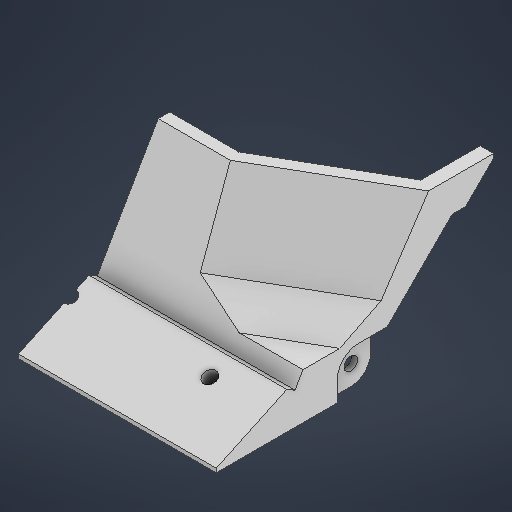
# Autodesk Inventor part: BodyFront
Saved by Autodesk Inventor 2027 (Build 310192000, 192)
## iProperties
Created: 2026-09-17
Part Number: BodyFront
Material: Všeobecné
Document SubType Name: Modeling
Designer: Vadim
Density: 1 g/cm^3
Appearance: Výchozí
Author: Vadim
Autodesk Inventor part; units mm, degrees
ref_plane "YZ Plane" through (0, 0, 0) normal (1, 0, 0) x (0, 1, 0)
ref_plane "XZ Plane" through (0, 0, 0) normal (0, 1, 0) x (-1, 0, 0)
ref_plane "XY Plane" through (0, 0, 0) normal (0, 0, 1) x (1, 0, 0)
sketch "Náčrt1" plane through (0, 0, 0) normal (1, 0, 0) x (0, 1, 0)
  circle A0 centre (0, 0) radius 5
  line L0 (5, 0) -> (5, -7)
  line L1 (5, -7) -> (21.5, -23.5)
  circle A1 centre (10.5, -45) radius 19.6
  circle A2 centre (8, -45) radius 19.6
  line L2 (21.5, -23.5) -> (21.5, -28.7778)
  line L3 (21.5, -28.2814) -> (29.5, -36.2814)
  circle A3 centre (10.5, -45) radius 18
  line L4 (28.5, -41.2264) -> (28.5, -45)
  line L5 (28.5, -41.2264) -> (28.1, -41.2264)
  line L6 (21.5, -26.8672) -> (29.5, -34.8672)
  line L7 (28.5, -41.2264) -> (29.5, -41.2264)
  line L8 (29.5, -41.2264) -> (29.5, -33.8672)
  line L9 (29.5, -33.8672) -> (28.5, -33.8672)
  line L10 (28.5, -33.8672) -> (28.5, -41.2264)
  line L11 (-5, 0) -> (-5, 35.5203)
  line L12 (7.6785, 17.8108) -> (-5, 45) construction
  line L13 (-5, 37.6648) -> (4.869, 16.5006) construction
  line L14 (4.869, 16.5006) -> (7.6785, 17.8108) construction
  line L15 (-5, 45) -> (-5, 37.6648) construction
  line L16 (-5, 35.5203) -> (-4, 35.5203)
  line L17 (-4, 35.5203) -> (4.2351, 17.8601)
  line L18 (29.5, 20.4961) -> (29.5, -33.8672)
  arc A4 (5.25, 0) -> (-5, 1.6008) centre (0, 0) ccw
  line L19 (5.25, 0) -> (5.25, -7.25)
  line L20 (4.2351, 17.8601) -> (3.0549, 15.816)
  line L21 (3.0549, 15.816) -> (29.5, 0.5479)
  line L22 (29.5, -2.3389) -> (-5, 17.5797)
  line L23 (5.25, 0) -> (5.25, 14.5486)
  line L24 (0, -5) -> (5, -5)
  line L25 (5, -5) -> (5.25, -5)
  line L26 (0, 5.25) -> (-5, 5.25)
  point P0 (5.25, 11.6619)
  dimension "d7" = 39.2
  dimension "d0" = 10
  dimension "d1" = 7
  dimension "d3" = 26.5
  dimension "d4" = 45
  dimension "d6" = 2.5
  dimension "d8" = 39.2
  dimension "d12" = 13
  dimension "d13" = 1.6
  dimension "d15" = 0.4
  dimension "d16" = 1
  dimension "d17" = 1
  dimension "d22" = 3.1
  dimension "d23" = 25
  dimension "d24" = 30
  dimension "d26" = 1
  dimension "d27" = 1.5
  dimension "d34" = 0.25
  dimension "d35" = 45
  dimension "d36" = 45
  dimension "d39" = 1.5
  dimension "d40" = 60
  dimension "d41" = 2.5
  constraints: 54 end point, 14 point on line, 8 point on circle, 7 parallel, 6 vertical, 5 perpendicular, 5 tangent, 4 centre point, 4 horizontal, 3 horizontal alignment, 2 collinear, 1 coincident, 4 other
  measures "d0" diameter of A0
  measures "d1" distance of L0.start L0.end
  measures "d3" horizontal distance of L1.end L11.start
  measures "d4" angle of L0 L1
  measures "d6" distance of A3.centre A2.centre
  measures "d8" diameter of A2
  measures "d12" horizontal distance of A2.centre L11.start
  measures "d15" distance of L4.start L5.end
  measures "d16" distance between parallel lines of L3 L6
  measures "d17" distance between parallel lines of L10 L8
  measures "d22" distance of L13.end L12.start
  measures "d23" angle of L12 L15
  measures "d24" distance of L12.start L12.end
  measures "d26" distance of L11.end L16.end
  measures "d27" distance from line of L14 L17.end
  measures "d34" radial gap between concentric circles of A0 A4
  measures "d35" vertical distance of point (0, 0) L12.end
  measures "d36" vertical distance of A2.centre point (0, 0)
  measures "d39" distance from line of L21 L13.end
  measures "d40" angle of L18 L21
  measures "d41" distance between parallel lines of L21 L22
extrude "Vysunutí1" add sketch "Náčrt1" against normal blind 49.5 contours L11 L16 L17 L20 L21 L23 L22 | L23 L21 L18 L22
extrude "Vysunutí2" add sketch "Náčrt1" against normal blind 3.35 contours L19 L23 L22 L18 L9 L6 L2 L1 | L11 L22 L23 A4 L26
extrude "Vysunutí6" add sketch "Náčrt1" against normal blind 3.35 contours A0 | L0 L24 A0 | A0 L11 A4 L19 L25 L0 | L11 L26 A4 | L11 L22 L23 A4 L26
ref_plane "Pracovní rovina1" through (-49.5, -4, 35.5203) normal (-0.8660254, 0, 0.5) x (0, 1, 0)
sketch "Náčrt2" plane through (-49.5, -4, 35.5203) normal (-0.8660254, 0, 0.5) x (0, 1, 0)
  line L0 (33.5, 24.1434) -> (9.5, 10.287)
  line L1 (9.5, 10.287) -> (9.5, 0.287)
  line L2 (9.5, 0.287) -> (15.6603, 10.9568)
  line L3 (15.6603, 10.9568) -> (33.5, 21.2566)
  line L4 (33.5, 21.2566) -> (33.5, 24.1434)
  line L5 (-1, -24.75) -> (-1, 0) projected
  line L6 (-1, 15.537) -> (-1, 0) projected
  line L7 (33.5, 5.537) -> (33.5, 30.287) projected
  line L8 (9.5, 0.287) -> (9.5, -10.1073)
  line L9 (33.5, 21.2566) -> (33.5, -4.0929)
  line L10 (33.5, -4.0929) -> (9.5, -10.1073)
  point P0 (4, 6.0115)
  dimension "d47" = 2.5
  dimension "d48" = 10.5
  dimension "d49" = 30
  dimension "d50" = 60
  dimension "d51" = 5.25
  dimension "d52" = 10
  constraints: 17 end point, 2 parallel, 2 vertical, 1 collinear, 1 point on line
  measures "d47" distance between parallel lines of L3 L0
  measures "d48" distance between parallel lines of L5 L1
  measures "d49" angle of L1 L2
  measures "d50" angle of L6 L0
  measures "d51" vertical distance of L0.end L6.start
  measures "d52" distance of L0.end L1.end
extrude "Vysunutí3" add sketch "Náčrt2" against normal up to surface contours L4 L3 L2 L1 L0 surface through (0, 12.25, 16.5907) normal (1, 0, 0)
extrude "Vysunutí4" cut sketch "Náčrt2" against normal up to surface surface through (0, 3.0549, 15.816) normal (0, 0.5, 0.8660254)
extrude "Vysunutí5" cut sketch "Náčrt2" against normal up to surface contours L7 L9 L10 L8 L2 L3 surface through (0, 12.25, 16.5907) normal (1, 0, 0)
extrude "Vysunutí10" cut sketch "Náčrt1" against normal blind 1.85 contours A0 | L0 L24 A0 | A0 L11 A4 L19 L25 L0 | L11 L26 A4
sketch "Náčrt6" plane through (-1.85, 0, 0) normal (1, 0, 0) x (0, 0, -1)
  arc A0 (0, -5) -> (5, 0) centre (0, 0) ccw projected
  constraints: 1 coincident
hole "Díra1" at (-1.85, 0, 0) direction (-1, 0, 0) diameter 3.35 end through all
sketch "Náčrt7" plane through (-28.5, 5.5, 11.5175) normal (0, -1, 0) x (1, 0, 0)
  line L0 (0, 0) -> (20, 0) projected
  line L1 (25.25, 0.1443) -> (25.2, 0.1443) projected
  line L2 (24.6, 0.1443) -> (24.6, -2.9445) projected
  line L3 (24.6, -2.9445) -> (24.6, -14.5204) projected
  line L4 (0, 0) -> (25.15, -14.5204) projected
  line L5 (25.6, -15.9349) -> (25.6, -2.6558)
  line L6 (25.6, -2.6558) -> (25.6, 1)
  line L7 (25.6, 1) -> (20, 1)
  line L8 (20, 1) -> (-3.7321, 1)
  line L9 (-3.7321, 1) -> (25.6, -15.9349)
  line L10 (25.15, -14.5204) -> (25.6, -14.7802)
  line L11 (0, 0) -> (-1.7321, 1)
  line L12 (28.5, 24.0027) -> (28.5, -6.2675) projected
  line L13 (28.5, -6.2675) -> (28.5, -11.5175) projected
  line L14 (28.5, 2.8969) -> (28.5, -11.5175)
  line L15 (28.5, -11.5175) -> (25.6, -11.5175)
  line L16 (28.5, 2.8969) -> (-3.7321, 2.8969)
  line L17 (-3.7321, 2.8969) -> (-3.7321, 1)
  point P0 (25.1, -2.9445)
  dimension "d79" = 1
  constraints: 22 end point, 5 point on line, 2 collinear, 2 perpendicular, 1 horizontal, 5 other
  measures "d79" distance between parallel lines of L4 L9
extrude "Vysunutí12" add sketch "Náčrt7" against normal blind 1 contours L11 L8 L7 L6 L5 L10 L4 | L8 L17 L16 L12 L13 L15 L5 L6 L7
sketch "Náčrt8" plane through (0, 0, 0) normal (1, 0, 0) x (0, 0, -1)
  line L0 (-15.816, 3.0549) -> (-17.8601, 4.2351) projected
  line L1 (-15.816, 3.0549) -> (-10.8842, 11.5969)
  line L2 (-10.8842, 11.5969) -> (-13.6098, 11.5969)
  line L3 (-13.6098, 11.5969) -> (-17.8601, 4.2351)
  line L4 (-17.8601, 4.2351) -> (-15.816, 3.0549)
  line L5 (0, 5.25) -> (7.25, 5.25) projected
  line L6 (7.25, 5.25) -> (23.5, 21.5) projected
  line L7 (23.5, 21.5) -> (26.8672, 21.5) projected
  line L8 (26.8672, 21.5) -> (33.8672, 28.5) projected
  line L9 (33.8672, 28.5) -> (33.8672, 29.5) projected
  line L10 (33.8672, 29.5) -> (17.6036, 29.5) projected
  line L11 (17.6036, 29.5) -> (5.7104, 11.6603) projected
  line L12 (5.7104, 11.6603) -> (-4.6101, 6.5) projected
  line L13 (-14.4145, 6.5) -> (-4.6101, 6.5) projected
  line L14 (-14.4145, 5.5) -> (-14.4145, 6.5) projected
  line L15 (-14.4043, 5.5) -> (-14.4145, 5.5) projected
  line L16 (-14.4043, 5.5) -> (-15.816, 3.0549) projected
  line L17 (-15.816, 3.0549) -> (-17.8601, 4.2351) projected
  line L18 (-17.8601, 4.2351) -> (-35.5203, -4) projected
  line L19 (-35.5203, -4) -> (-35.5203, -5) projected
  line L20 (-35.5203, -5) -> (-5.25, -5) projected
  line L21 (-5.25, -5) -> (-5.25, 0) projected
  arc A0 (0, 5.25) -> (-5.25, 0) centre (0, 0) ccw projected
  line L22 (-25.2608, 3.5425) -> (-22.5419, 4.8104) construction
  line L23 (-22.5419, 4.8104) -> (-20.1118, -0.4009) construction
  line L24 (-20.1118, -0.4009) -> (-22.8308, -1.6688) construction
  line L25 (-22.8308, -1.6688) -> (-25.2608, 3.5425) construction
  line L26 (-22.8308, -1.6688) -> (-23.9191, -4.6588) construction
  line L27 (-23.9191, -4.6588) -> (-17.1217, -1.4892) construction
  line L28 (-17.1217, -1.4892) -> (-20.1118, -0.4009) construction
  line L29 (-23.9013, 4.1764) -> (-20.5204, -3.074) construction
  line L30 (-35.5203, -5) -> (-37.6648, -5)
  line L31 (-37.6648, -5) -> (-35.5203, -4)
  line L32 (-17.8601, 4.2351) -> (-16.5006, 4.869)
  line L33 (-35.5203, -5) -> (-24.0203, -5)
  line L34 (-35.5203, -5) -> (-5.25, -5) projected
  line L35 (-11.5175, 5.5) -> (-17.5797, -5) projected
  line L36 (-24.0203, -5) -> (-15.207, -0.8903)
  point P0 (-11.6619, 5.25)
  dimension "d84" = 7.5
  dimension "d85" = 3
  dimension "d86" = 8
  dimension "d87" = 2.5
  dimension "d89" = 1.5
  dimension "d90" = 5.5
  dimension "d92" = 5.5
  dimension "d93" = 11.5
  dimension "d94" = 25
  constraints: 34 end point, 4 parallel, 4 perpendicular, 2 collinear, 2 horizontal, 2 midpoint, 2 point on line, 1 other
  measures "d84" distance of L26.end L27.end
  measures "d85" distance between parallel lines of L25 L23
  measures "d86" distance between parallel lines of L27 L22
  measures "d87" distance between parallel lines of L18 L22
  measures "d89" distance from line of L16 L32.end
  measures "d90" distance from line of L23 L32.end
  measures "d92" distance from line of L0.end L29
  measures "d93" distance of L19.end L33.end
  measures "d94" angle of L20 L36
extrude "Vysunutí13" cut sketch "Náčrt8" against normal up to surface (49.5 mm away) contours L0 L3 L2 L1 L13 L14 L15 | L15 L14 L13 L1
sketch "Náčrt9" plane through (-49.5, 0, 0) normal (-1, 0, 0) x (0, 0, 1)
  line L0 (35.5203, -4) -> (17.8601, 4.2351) projected
  line L1 (17.8601, 4.2351) -> (15.816, 3.0549) projected
  line L2 (15.816, 3.0549) -> (0.5479, 29.5) projected
  line L3 (0.5479, 29.5) -> (-2.3389, 29.5) projected
  line L4 (-2.3389, 29.5) -> (17.5797, -5) projected
  line L5 (17.5797, -5) -> (35.5203, -5) projected
  line L6 (35.5203, -5) -> (35.5203, -4) projected
  line L7 (35.5203, -5) -> (24.0203, -5)
  line L8 (24.0203, -5) -> (15.207, -0.8903)
  point P0 (0, 0)
  dimension "d95" = 11.5
  dimension "d96" = 25
  constraints: 4 end point, 2 point on line
  measures "d95" distance of L5.end L7.end
  measures "d96" angle of L5 L8
extrude "Vysunutí14" cut sketch "Náčrt9" against normal up to surface (46.15 mm away) contours L5 L4 L8
sketch "Náčrt11" plane through (-49.5, -5, 24.0203) normal (0, -0.9063078, -0.4226183) x (1, 0, 0)
  line L0 (0, -9.7244) -> (0, 0) projected
  line L1 (46.15, -9.7244) -> (0, -9.7244) projected
  point P0 (49.5, -23.8828)
  point P1 (0, -4.2244)
  point P2 (35, -4.2244)
  dimension "d110" = 0
  dimension "d111" = 5.5
  dimension "d112" = 5.5
  dimension "d113" = 35
  measures "d110" distance from line of L0 point (0, -4.224)
  measures "d111" distance from line of L1 point (0, -4.224)
  measures "d112" distance from line of L1 point (35, -4.224)
  measures "d113" distance from line of L0 point (35, -4.224)
hole "Díra2" at (-49.5, -3.2147, 20.1917) at (-14.5, -3.2147, 20.1917) direction (0, 0.9063078, 0.4226183) diameter 3.35 end through all countersink diameter 7.5 countersink angle 90
equation "\"d8\" = d7"
